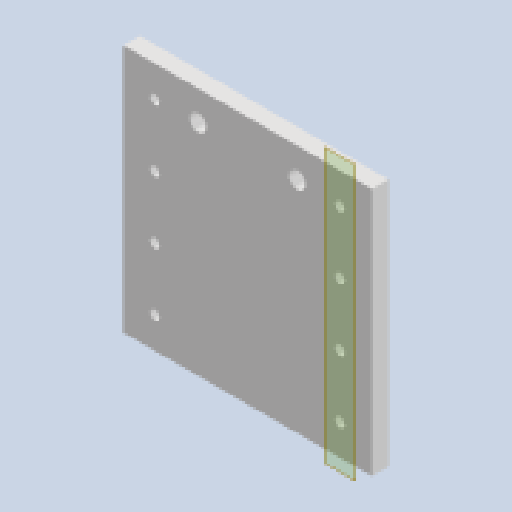
# Autodesk Inventor part: деталь которая двигает
Saved by Autodesk Inventor 2024.2 (Build 282272000, 272)
## iProperties
Created: 2025-11-27
Part Number: деталь которая двигает
Material: Типовые
Document SubType Name: Modeling
Designer: katya_notebook
Density: 1 g/cm^3
Appearance: По умолчанию
Author: katya_notebook
Autodesk Inventor part; units mm, degrees
ref_plane "YZ Plane" through (0, 0, 0) normal (1, 0, 0) x (0, 1, 0)
ref_plane "XZ Plane" through (0, 0, 0) normal (0, 1, 0) x (-1, 0, 0)
ref_plane "XY Plane" through (0, 0, 0) normal (0, 0, 1) x (1, 0, 0)
ref_plane "РабПлоскость2" through (101.7859, 42.6575, -2.4) normal (0, 0, -1) x (-1, 0, 0)
sketch "Эскиз2" plane through (101.7859, 42.6575, -2.4) normal (0, 0, -1) x (-1, 0, 0)
  line L0 (-6.6, -87.5) -> (0, -87.5) projected
  line L1 (0, -27.5) -> (0, -87.5) projected
  line L2 (0, -27.5) -> (-6.6, -27.5) projected
  line L3 (-6.6, -27.5) -> (-6.6, -87.5) projected
  circle A0 centre (-3.3, -35) radius 2.3 projected
  circle A1 centre (-3.3, -50) radius 2.3 projected
  circle A2 centre (-3.3, -65) radius 2.3 projected
  circle A3 centre (-3.3, -80) radius 2.3 projected
  line L4 (38, -87.5) -> (44.6, -87.5) projected
  line L5 (44.6, -27.5) -> (44.6, -87.5) projected
  line L6 (44.6, -27.5) -> (38, -27.5) projected
  line L7 (38, -27.5) -> (38, -87.5) projected
  circle A4 centre (41.3, -35) radius 2.3 projected
  circle A5 centre (41.3, -50) radius 2.3 projected
  circle A6 centre (41.3, -65) radius 2.3 projected
  circle A7 centre (41.3, -80) radius 2.3 projected
  line L8 (-11.0784, -27.5) -> (48.9216, -27.5)
  line L9 (48.9216, -27.5) -> (48.9216, -87.5)
  line L10 (48.9216, -87.5) -> (-11.0784, -87.5)
  line L11 (-11.0784, -87.5) -> (-11.0784, -27.5)
  line L12 (18.9216, -50) -> (18.9216, -69.7785)
  circle A8 centre (-3.3, -35) radius 1.2 projected
  circle A9 centre (-3.3, -50) radius 1.2 projected
  circle A10 centre (-3.3, -65) radius 1.2 projected
  circle A11 centre (-3.3, -80) radius 1.2 projected
  circle A12 centre (41.3, -80) radius 1.2 projected
  circle A13 centre (41.3, -65) radius 1.2 projected
  circle A14 centre (41.3, -50) radius 1.2 projected
  circle A15 centre (41.3, -35) radius 2.1 projected
  circle A16 centre (41.3, -35) radius 1.2 projected
  point P0 (101.7859, -42.6575)
  point P1 (0, -87.5)
  point P2 (0, -27.5)
  point P3 (-6.6, -27.5)
  dimension "d3" = 60
  dimension "d4" = 60
  dimension "d5" = 30
  constraints: 10 end point, 2 parallel, 2 vertical, 1 horizontal, 1 perpendicular
  measures "d3" distance of L8.start L8.end
  measures "d4" distance of L8.end L9.end
  measures "d5" distance between parallel lines of L11 L12
extrude "Выдавливание2" add sketch "Эскиз2" along normal blind 4 contours L3 L2 L1 L0 | L10 L11 L8 L3 | L1 L8 L7 L10 | L7 L6 L5 L4 | L5 L8 L9 L10 | A0 | A1 | A2 | A3 | A4 | A5 | A6 | A7 | A15
sketch "Эскиз3" plane through (101.7859, 42.6575, -6.4) normal (0, 0, -1) x (-1, 0, 0)
  circle A0 centre (7, -34.5989) radius 2 projected
  circle A1 centre (31, -34.5989) radius 2 projected
  point P0 (101.7859, -42.6575)
extrude "Выдавливание3" cut sketch "Эскиз3" against normal blind 10
